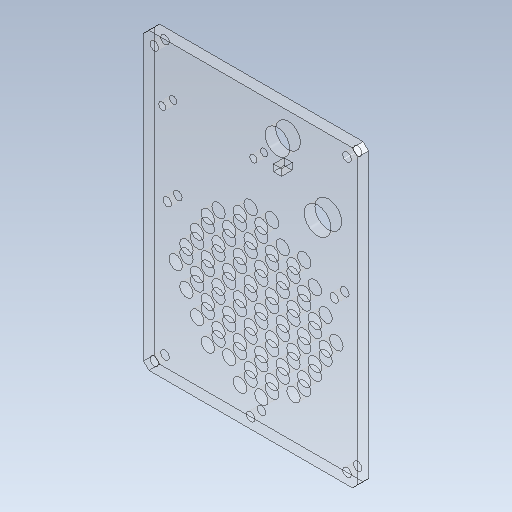
# Autodesk Inventor part: front_pannel
Saved by Autodesk Inventor 2026.1 (Build 301233020, 233B)
## iProperties
Created: 2026-08-15
Part Number: front_pannel
Material: PMMA プラスチック
Document SubType Name: Modeling
Designer: ug_nd
Density: 1.188 g/cm^3
Appearance: ポリカーボネート - クリア
Author: ug_nd
Autodesk Inventor part; units mm, degrees
ref_plane "YZ Plane" through (0, 0, 0) normal (1, 0, 0) x (0, 1, 0)
ref_plane "XZ Plane" through (0, 0, 0) normal (0, 1, 0) x (-1, 0, 0)
ref_plane "XY Plane" through (0, 0, 0) normal (0, 0, 1) x (1, 0, 0)
sketch "スケッチ1" plane through (0, 0, 0) normal (0, 0, 1) x (1, 0, 0)
  line L0 (-40, -55) -> (40, -55)
  line L1 (40, -55) -> (40, 55)
  line L2 (40, 55) -> (-40, 55)
  line L3 (-40, 55) -> (-40, -55)
  line L4 (-40, -55) -> (40, 55) construction
  line L5 (40, -55) -> (-40, 55) construction
  circle A0 centre (10, 43) radius 4.6
  circle A1 centre (25, 25) radius 5
  circle A2 centre (25, 25) radius 12.5 construction
  circle A3 centre (10, 43) radius 8.25 construction
  line L6 (0, -77) -> (0, 77) construction
  circle A4 centre (0, -15) radius 32.75 construction
  line L7 (-36, 20) -> (4, 20) construction
  line L8 (4, 20) -> (4, 36) construction
  line L9 (4, 36) -> (-36, 36) construction
  line L10 (-36, 36) -> (-36, 20) construction
  line L11 (-36, 20) -> (4, 36) construction
  line L12 (4, 20) -> (-36, 36) construction
  line L13 (13.4369, 50.5) -> (21.75, 50.5) construction
  line L14 (21.75, 50.5) -> (21.75, 35.5) construction
  line L15 (21.75, 35.5) -> (13.4369, 35.5) construction
  line L16 (8.5, 32.5) -> (8.5, 35)
  line L17 (8.5, 35) -> (11.5, 35)
  line L18 (11.5, 35) -> (11.5, 32.5)
  line L19 (8.5, 32.5) -> (11.5, 32.5)
  line L20 (8.5, 35) -> (11.5, 32.5) construction
  line L21 (11.5, 35) -> (8.5, 32.5) construction
  line L22 (0, -15) -> (28.3623, 1.375) construction
  line L23 (0, -15) -> (-28.3623, 1.375) construction
  circle A5 centre (0, -15) radius 36 construction
  circle A6 centre (31.1769, 3) radius 1.6
  circle A7 centre (-31.1769, 3) radius 1.6
  circle A8 centre (0, -51) radius 1.6
  line L24 (-32.75, -15) -> (32.75, -15) construction
  circle A9 centre (-4, -15) radius 2.5
  circle A10 centre (0, -8.0718) radius 2.5
  circle A11 centre (4, -15) radius 2.5
  circle A12 centre (8, -8.0718) radius 2.5
  circle A13 centre (-12, -15) radius 2.5
  circle A14 centre (-8, -8.0718) radius 2.5
  circle A15 centre (12, -15) radius 2.5
  circle A16 centre (16, -8.0718) radius 2.5
  circle A17 centre (-20, -15) radius 2.5
  circle A18 centre (-16, -8.0718) radius 2.5
  circle A19 centre (20, -15) radius 2.5
  circle A20 centre (24, -8.0718) radius 2.5
  circle A21 centre (-4, -1.1436) radius 2.5
  circle A22 centre (0, 5.7846) radius 2.5
  circle A23 centre (4, -1.1436) radius 2.5
  circle A24 centre (8, 5.7846) radius 2.5
  circle A25 centre (-12, -1.1436) radius 2.5
  circle A26 centre (-8, 5.7846) radius 2.5
  circle A27 centre (12, -1.1436) radius 2.5
  circle A28 centre (16, 5.7846) radius 2.5
  circle A29 centre (-20, -1.1436) radius 2.5
  circle A30 centre (-16, 5.7846) radius 2.5
  circle A31 centre (20, -1.1436) radius 2.5
  circle A32 centre (24, 5.7846) radius 2.5 construction
  circle A33 centre (-4, -28.8564) radius 2.5
  circle A34 centre (0, -21.9282) radius 2.5
  circle A35 centre (4, -28.8564) radius 2.5
  circle A36 centre (8, -21.9282) radius 2.5
  circle A37 centre (-12, -28.8564) radius 2.5
  circle A38 centre (-8, -21.9282) radius 2.5
  circle A39 centre (12, -28.8564) radius 2.5
  circle A40 centre (16, -21.9282) radius 2.5
  circle A41 centre (-20, -28.8564) radius 2.5
  circle A42 centre (-16, -21.9282) radius 2.5
  circle A43 centre (20, -28.8564) radius 2.5
  circle A44 centre (24, -21.9282) radius 2.5
  circle A45 centre (-4, 12.7128) radius 2.5
  circle A46 centre (0, 19.641) radius 2.5 construction
  circle A47 centre (4, 12.7128) radius 2.5
  circle A48 centre (8, 19.641) radius 2.5 construction
  circle A49 centre (-12, 12.7128) radius 2.5 construction
  circle A50 centre (-8, 19.641) radius 2.5 construction
  circle A51 centre (12, 12.7128) radius 2.5 construction
  circle A52 centre (16, 19.641) radius 2.5 construction
  circle A53 centre (-20, 12.7128) radius 2.5 construction
  circle A54 centre (-16, 19.641) radius 2.5 construction
  circle A55 centre (20, 12.7128) radius 2.5 construction
  circle A56 centre (24, 19.641) radius 2.5 construction
  circle A57 centre (-4, -42.7128) radius 2.5
  circle A58 centre (0, -35.7846) radius 2.5
  circle A59 centre (4, -42.7128) radius 2.5
  circle A60 centre (8, -35.7846) radius 2.5
  circle A61 centre (-12, -42.7128) radius 2.5 construction
  circle A62 centre (-8, -35.7846) radius 2.5
  circle A63 centre (12, -42.7128) radius 2.5 construction
  circle A64 centre (16, -35.7846) radius 2.5
  circle A65 centre (-20, -42.7128) radius 2.5 construction
  circle A66 centre (-16, -35.7846) radius 2.5
  circle A67 centre (20, -42.7128) radius 2.5 construction
  circle A68 centre (24, -35.7846) radius 2.5 construction
  circle A69 centre (0, -15) radius 30 construction
  circle A70 centre (-28, -15) radius 2.5
  circle A71 centre (-24, -8.0718) radius 2.5
  circle A72 centre (-28, -1.1436) radius 2.5 construction
  circle A73 centre (-24, 5.7846) radius 2.5 construction
  circle A74 centre (-28, -28.8564) radius 2.5 construction
  circle A75 centre (-24, -21.9282) radius 2.5
  circle A76 centre (-28, 12.7128) radius 2.5 construction
  circle A77 centre (-24, 19.641) radius 2.5 construction
  circle A78 centre (-28, -42.7128) radius 2.5 construction
  circle A79 centre (-24, -35.7846) radius 2.5 construction
  circle A80 centre (28, -15) radius 2.5
  circle A81 centre (32, -8.0718) radius 2.5 construction
  circle A82 centre (28, -1.1436) radius 2.5 construction
  circle A83 centre (32, 5.7846) radius 2.5 construction
  circle A84 centre (28, -28.8564) radius 2.5 construction
  circle A85 centre (32, -21.9282) radius 2.5 construction
  circle A86 centre (28, 12.7128) radius 2.5 construction
  circle A87 centre (32, 19.641) radius 2.5 construction
  circle A88 centre (28, -42.7128) radius 2.5 construction
  circle A89 centre (32, -35.7846) radius 2.5 construction
  circle A90 centre (-33, 33) radius 1.35
  circle A91 centre (1, 33) radius 1.35
  point P0 (0, 0)
  point P1 (-16, 28)
  point P2 (10, 33.75)
  point P3 (10, 33.75)
  dimension "d32" = 72
  dimension "d0" = 110
  dimension "d1" = 80
  dimension "d2" = 12
  dimension "d3" = 9.2
  dimension "d5" = 30
  dimension "d6" = 15
  dimension "d7" = 30
  dimension "d8" = 25
  dimension "d9" = 10
  dimension "d10" = 25
  dimension "d11" = 16.5
  dimension "d12" = 65.5
  dimension "d15" = 15
  dimension "d16" = 40
  dimension "d17" = 16
  dimension "d19" = 4
  dimension "d20" = 35
  dimension "d21" = 40
  dimension "d22" = 58
  dimension "d23" = 15
  dimension "d24" = 11.75
  dimension "d27" = 3
  dimension "d29" = 8
  dimension "d30" = 2.5
  dimension "d31" = 120
  dimension "d33" = 3.2
  dimension "d36" = 360
  dimension "d38" = 5
  dimension "d39" = 8
  dimension "d43" = 8
  dimension "d46" = 13.8564
  dimension "d49" = 8
  dimension "d50" = 60
  dimension "d51" = 2.7
  dimension "d52" = 3
  dimension "d53" = 3
  dimension "d54" = 3
  dimension "d55" = 3
  dimension "d61" = 10
  constraints: 91 centre point, 48 end point, 8 horizontal, 7 midpoint, 5 parallel, 5 point on circle, 4 coincident, 4 point on line, 4 vertical, 2 equal radius, 2 perpendicular, 2 symmetric about line, 1 horizontal alignment, 1 vertical alignment, 166 other
  measures "d0" distance of L0.end L1.end
  measures "d1" distance of L1.end L2.end
  measures "d2" distance from line of A0.centre L2
  measures "d3" diameter of A0
  measures "d5" distance from line of L1 A0.centre
  measures "d6" distance from line of L1 A1.centre
  measures "d7" distance from line of A1.centre L2
  measures "d8" diameter of A2
  measures "d9" horizontal distance of A0.centre point (0, 0)
  measures "d10" horizontal distance of A1.centre point (0, 0)
  measures "d11" diameter of A3
  measures "d12" diameter of A4
  measures "d15" distance of point (0, 0) L22.start
  measures "d16" distance of L8.end L9.end
  measures "d17" distance of L9.end L7.start
  measures "d19" distance between parallel lines of L3 L10
  measures "d20" distance from line of L22.start L7
  measures "d21" vertical distance of L22.start A2.centre
  measures "d22" vertical distance of L22.start A0.centre
  measures "d23" distance between parallel lines of L15 L13
  measures "d24" distance from line of L14 A0.centre
  measures "d27" distance between parallel lines of L18 L16
  measures "d29" distance from line of L17 A0.centre
  measures "d30" distance of L17.end L18.end
  measures "d31" angle of L22 L23
  measures "d33" diameter of A6
  measures "d38" diameter of A9
  measures "d39" distance of A9.centre A10.centre
  measures "d43" distance of A9.centre A11.centre
  measures "d46" distance of A9.centre A21.centre
  measures "d49" distance of A10.centre A21.centre
  measures "d50" diameter of A69
  measures "d51" diameter of A90
  measures "d52" distance from line of L9 A90.centre
  measures "d53" distance from line of L10 A90.centre
  measures "d54" distance from line of L8 A91.centre
  measures "d55" distance from line of L9 A91.centre
  measures "d61" diameter of A1
extrude "押し出し1" add sketch "スケッチ1" along normal blind 4
chamfer "面取り1" distance 2 angle 45 4 edges at (40, 55, 2) (-40, 55, 2) (-40, -55, 2) (40, -55, 2)
sketch "スケッチ2" plane through (0, 0, 4) normal (0, 0, 1) x (1, 0, 0)
  line L0 (36, -51) -> (-36, -51) construction
  line L1 (-36, -51) -> (-36, 51) construction
  line L2 (-36, 51) -> (36, 51) construction
  line L3 (36, 51) -> (36, -51) construction
  line L4 (36, -51) -> (-36, 51) construction
  line L5 (-36, -51) -> (36, 51) construction
  circle A0 centre (-36, 51) radius 1.6
  circle A1 centre (36, 51) radius 1.6
  circle A2 centre (-36, -51) radius 1.6
  circle A3 centre (36, -51) radius 1.6
  line L6 (-40, 53) -> (-40, -53) construction
  line L7 (38, 55) -> (-38, 55) construction
  point P0 (0, 0)
  dimension "d62" = 3.2
  dimension "d63" = 4
  dimension "d64" = 4
  constraints: 12 end point, 4 centre point, 4 coincident, 3 equal radius, 2 midpoint, 2 parallel, 1 horizontal, 1 perpendicular
  measures "d62" diameter of A0
  measures "d63" distance between parallel lines of L6 L1
  measures "d64" distance between parallel lines of L7 L2
extrude "押し出し2" cut sketch "スケッチ2" against normal through all
equation "\"d39\" = d43"
equation "\"d49\" = d43"
equation "\"d64\" = d63"
